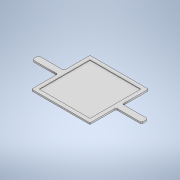
# Autodesk Inventor part: MouldBase20
Saved by Autodesk Inventor 2020.3 (Build 243373010, 373A)
## iProperties
Created: 2020-10-26
Part Number: MouldBase20
Material: Generic
Document SubType Name: Modeling
Designer: Naude Conradie
Density: 1 g/cm^3
Appearance: Default
Author: Naude Conradie
Autodesk Inventor part; units mm, degrees
ref_plane "YZ Plane" through (0, 0, 0) normal (1, 0, 0) x (0, 1, 0)
ref_plane "XZ Plane" through (0, 0, 0) normal (0, 1, 0) x (-1, 0, 0)
ref_plane "XY Plane" through (0, 0, 0) normal (0, 0, 1) x (1, 0, 0)
sketch "Sketch1" plane through (0, 0, 0) normal (0, 1, 0) x (-1, 0, 0)
  line L0 (0, 0) -> (230, 0)
  line L1 (230, 0) -> (230, -230)
  line L2 (230, -230) -> (0, -230)
  line L3 (0, -230) -> (0, 0)
  dimension "d0" = 230
  dimension "d1" = 230
  constraints: 8 end point, 2 parallel, 1 horizontal, 1 perpendicular
  measures "d0" distance of L1.end L2.end
  measures "d1" distance of L0.end L1.end
extrude "Extrusion1" add sketch "Sketch1" along normal blind 6
sketch "Sketch2" plane through (0, 6, 0) normal (0, 1, 0) x (1, 0, 0)
  line L0 (-215, 215) -> (-15, 215)
  line L1 (-15, 215) -> (-15, 15)
  line L2 (-15, 15) -> (-215, 15)
  line L3 (-215, 15) -> (-215, 215)
  line L4 (-230, 230) -> (-230, 0) projected
  point P0 (0, 0)
  dimension "d4" = 200
  dimension "d5" = 200
  dimension "d6" = 15
  dimension "d7" = 15
  constraints: 8 end point, 2 parallel, 1 horizontal, 1 perpendicular
  measures "d4" distance of L1.end L2.end
  measures "d5" distance of L0.end L1.end
  measures "d6" distance from line of L4 L0.start
  measures "d7" distance from line of L0 L4.start
extrude "Extrusion2" cut sketch "Sketch2" against normal blind 2
chamfer "Chamfer1" distance 2 angle 45 4 edges at (-230, 3, 0) (-230, 3, -230) (0, 3, -230) (0, 3, 0)
sketch "Sketch3" plane through (0, 0, -2) normal (1, 0, 0) x (0, 0, -1)
  line L0 (0, 6) -> (226, 6) projected
  line L1 (13, 6) -> (213, 6) projected
  line L2 (100.5, 0) -> (125.5, 0)
  line L3 (125.5, 0) -> (125.5, 6)
  line L4 (125.5, 6) -> (100.5, 6)
  line L5 (100.5, 6) -> (100.5, 0)
  point P0 (-2, 0)
  dimension "d13" = 25
  dimension "d14" = 102.5
  constraints: 8 end point, 2 parallel, 1 horizontal, 1 perpendicular, 1 point on line
  measures "d13" distance of L4.end L3.end
  measures "d14" distance of point (-2, 0) L2.start
extrude "Extrusion3" add sketch "Sketch3" along normal blind 100
fillet "Fillet1" radius 5 2 edges at (0, 3, -102.5) (0, 3, -127.5)
chamfer "Chamfer2" distance 5 angle 45 2 edges at (100, 3, -102.5) (100, 3, -127.5)
sketch "Sketch4" plane through (-230, 0, -228) normal (-1, 0, 0) x (0, 0, 1)
  line L0 (0, 6) -> (226, 6) projected
  line L1 (13, 6) -> (213, 6) projected
  line L2 (100.5, 0) -> (125.5, 0)
  line L3 (125.5, 0) -> (125.5, 6)
  line L4 (125.5, 6) -> (100.5, 6)
  line L5 (100.5, 6) -> (100.5, 0)
  line L6 (-2, 6) -> (-2, 0) projected
  point P0 (228, 0)
  dimension "d21" = 25
  dimension "d22" = 102.5
  constraints: 8 end point, 2 parallel, 1 horizontal, 1 perpendicular, 1 point on line
  measures "d21" distance of L4.end L3.end
  measures "d22" distance from line of L6 L2.start
extrude "Extrusion4" add sketch "Sketch4" along normal blind 100
fillet "Fillet2" radius 5 2 edges at (-230, 3, -102.5) (-230, 3, -127.5)
chamfer "Chamfer3" distance 5 angle 45 2 edges at (-330, 3, -102.5) (-330, 3, -127.5)
body "Solid1"
